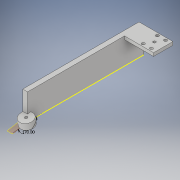
# Autodesk Inventor part: WheelIntakeMotorMount
Saved by Autodesk Inventor 2017 (Build 210142000, 142)
## iProperties
Created: 2017-11-15
Part Number: WheelIntakeMotorMount
Material: Generic
Document SubType Name: Modeling
Designer: User
Density: 1 g/cm^3
Appearance: Default
Author: User
Autodesk Inventor part; units mm, degrees
ref_plane "YZ Plane" through (0, 0, 0) normal (1, 0, 0) x (0, 1, 0)
ref_plane "XZ Plane" through (0, 0, 0) normal (0, 1, 0) x (-1, 0, 0)
ref_plane "XY Plane" through (0, 0, 0) normal (0, 0, 1) x (1, 0, 0)
sketch "Sketch2" plane through (0, 0, 0) normal (1, 0, 0) x (0, 1, 0)
  line L0 (0, 0) -> (25.4, 0)
  line L1 (25.4, 0) -> (25.4, -114.3)
  line L2 (25.4, -114.3) -> (0, -114.3)
  line L3 (0, -114.3) -> (0, 0)
  dimension "d6" = 25.4
  dimension "d7" = 114.3
  constraints: 8 end point, 2 parallel, 1 horizontal, 1 perpendicular
  measures "d6" distance of L1.end L2.end
  measures "d7" distance of L0.end L1.end
extrude "Extrusion2" add sketch "Sketch2" along normal blind 4.7625
sketch "Sketch3" plane through (4.7625, 0, 0) normal (1, 0, 0) x (0, 0, -1)
  line L0 (0, 0) -> (114.3, 0) projected
  line L1 (0, 0) -> (-14.429, -2.5442)
  line L2 (0, 0) -> (14.6516, 0) construction
  dimension "d10" = 170
  constraints: 4 end point, 1 equal length, 1 horizontal
  measures "d10" angle of L1 L2
ref_plane "Work Plane1" through (4.7625, -2.5442, 14.429) normal (0, 0.9848078, 0.1736482) x (0, 0.1736482, -0.9848078)
sketch "Sketch4" plane through (4.7625, -2.5442, 14.429) normal (0, 0.9848078, 0.1736482) x (0, 0.1736482, -0.9848078)
  line L0 (127.2151, 4.7625) -> (14.6516, 4.7625) projected
  line L1 (127.2151, 4.7625) -> (127.2151, 0) projected
  line L2 (14.6516, 0) -> (127.2151, 0) projected
  line L3 (14.6516, 4.7625) -> (14.6516, 0) projected
  line L4 (14.6516, 4.7625) -> (14.6516, 0)
  circle A0 centre (12.7466, -1.5875) radius 6.35
  dimension "d28" = 12.7
  dimension "d29" = 4.7625
  dimension "d30" = 1.5875
  dimension "d40" = 1.905
  constraints: 2 end point, 1 centre point, 1 collinear
  measures "d28" diameter of A0
  measures "d29" distance of L0.end L2.start
  measures "d30" distance from line of L2 A0.centre
  measures "d40" distance from line of A0.centre L3
sketch "Sketch5" plane through (0, 25.4, 0) normal (0, 1, 0) x (1, 0, 0)
  line L0 (0, 0) -> (0, 114.3) projected
  line L1 (0, 0) -> (4.7625, 0) projected
  line L2 (4.7625, 114.3) -> (4.7625, 0) projected
  line L3 (0, 114.3) -> (4.7625, 114.3) projected
  line L4 (0, 114.3) -> (0, 0) projected
  line L5 (0, 114.3) -> (33.3375, 114.3)
  line L6 (33.3375, 114.3) -> (33.3375, 95.25)
  line L7 (33.3375, 95.25) -> (0, 95.25)
  line L8 (0, 95.25) -> (0, 114.3)
  dimension "d47" = 33.3375
  dimension "d48" = 4.7625
  dimension "d49" = 19.05
  constraints: 8 end point, 2 parallel, 1 horizontal, 1 perpendicular
  measures "d47" distance of L6.end L7.end
  measures "d48" distance of L0.end L2.start
  measures "d49" distance of L5.end L6.end
extrude "Extrusion4" add sketch "Sketch5" against normal blind 3.175 contours L0 L3 L2 L7 | L2 L5 L6 L7
extrude "Extrusion6" add sketch "Sketch4" along normal blind 6.35 contours A0 L2 L3 | L3 L2 A0
sketch "Sketch10" plane through (0, 0, 0) normal (-1, 0, 0) x (0, 0, 1)
  line L0 (0, 25.4) -> (-114.3, 25.4) projected
  line L1 (-114.3, 25.4) -> (-114.3, 0) projected
  line L2 (-114.3, 0) -> (0, 0) projected
  line L3 (0, 0) -> (0, 25.4) projected
  line L4 (-3.0762, 6.9904) -> (-4.1789, 0.7369) projected
  line L5 (0, 6.448) -> (-3.0762, 6.9904) projected
  line L6 (0, 0) -> (0, 6.448) projected
  line L7 (-4.1789, 0.7369) -> (0, 0) projected
  line L8 (9.2323, 4.8201) -> (-3.2748, 7.0254) projected
  line L9 (8.1296, -1.4335) -> (9.2323, 4.8201) projected
  line L10 (3.078, 5.9052) -> (1.5105, -2.9848)
  line L11 (3.078, 5.9052) -> (12.1052, 5.9052) construction
  line L12 (-114.3, 0) -> (0, 0) projected
  line L13 (3.078, 5.9052) -> (0, 6.448)
  line L14 (0, 0) -> (0, 25.4) projected
  line L15 (0, 0) -> (0, 6.448)
  line L16 (0, 0) -> (1.9753, -0.3483)
  line L17 (5.253, -0.9262) -> (-1.5008, 0.2646) projected
  line L18 (0, 0) -> (4.9253, -0.8685)
  point P0 (-1.1172, 0.197)
  dimension "d41" = 12.3085
  dimension "d42" = 6.1542
  dimension "d43" = 100
  dimension "d44" = 8.89
  constraints: 12 end point, 4 point on line, 2 collinear, 1 equal length, 1 horizontal
  measures "d41" horizontal distance of L8.start L4.start
  measures "d42" horizontal distance of L8.start L10.start
  measures "d43" angle of L10 L11
  measures "d44" vertical distance of L10.start L10.end
extrude "Extrusion9" add sketch "Sketch10" against normal blind 2.54
sketch "Sketch11" plane through (0, 25.4, 0) normal (0, 1, 0) x (1, 0, 0)
  line L0 (0, 0) -> (4.7625, 0) projected
  line L1 (4.7625, 95.25) -> (4.7625, 0) projected
  line L2 (4.7625, 95.25) -> (33.3375, 95.25) projected
  line L3 (33.3375, 95.25) -> (33.3375, 114.3) projected
  line L4 (0, 114.3) -> (33.3375, 114.3) projected
  line L5 (0, 0) -> (0, 114.3) projected
  circle A0 centre (24.6375, 104.775) radius 8
  line L6 (20.6375, 111.7032) -> (28.6375, 111.7032)
  line L7 (28.6375, 111.7032) -> (28.6375, 97.8468)
  line L8 (28.6375, 97.8468) -> (20.6375, 97.8468)
  line L9 (20.6375, 97.8468) -> (20.6375, 111.7032)
  point P0 (0, 0)
  dimension "d50" = 16
  dimension "d53" = 19.05
  dimension "d54" = 28.575
  dimension "d55" = 9.525
  dimension "d56" = 8
  dimension "d57" = 4
  dimension "d58" = 15.875
  constraints: 8 end point, 4 coincident, 2 parallel, 2 point on circle, 1 centre point, 1 horizontal, 1 perpendicular
  measures "d50" diameter of A0
  measures "d53" distance of L2.end L3.end
  measures "d54" distance of L1.start L2.end
  measures "d55" distance from line of L4 A0.centre
  measures "d56" distance of L6.start L6.end
  measures "d57" distance from line of A0.centre L9
  measures "d58" distance from line of L1 point (20.637, 97.847)
hole "Hole1" at (20.6375, 25.4, -111.7032) at (28.6375, 25.4, -111.7032) at (28.6375, 25.4, -97.8468) at (20.6375, 25.4, -97.8468) direction (0, -1, 0) diameter 2.921 end through all
sketch "Sketch12" plane through (0, 25.4, 0) normal (0, 1, 0) x (1, 0, 0)
  circle A0 centre (28.6375, 97.8468) radius 1.4605 projected
  circle A1 centre (20.6375, 111.7032) radius 1.4605 projected
  circle A2 centre (28.6375, 111.7032) radius 1.4605 projected
  circle A3 centre (20.6375, 97.8468) radius 1.4605 projected
  line L0 (0, 0) -> (4.7625, 0) projected
  line L1 (4.7625, 95.25) -> (4.7625, 0) projected
  line L2 (4.7625, 95.25) -> (33.3375, 95.25) projected
  line L3 (33.3375, 95.25) -> (33.3375, 114.3) projected
  line L4 (0, 114.3) -> (33.3375, 114.3) projected
  line L5 (0, 0) -> (0, 114.3) projected
  circle A4 centre (28.6375, 97.8468) radius 1.4605 projected
  arc A5 (20.6375, 111.7032) -> (28.6375, 111.7032) centre (24.6375, 104.775) ccw
  point P0 (0, 0)
  constraints: 3 point on circle, 1 centre point
hole "Hole2" at (24.6375, 25.4, -104.775) direction (0, -1, 0) diameter 2.54 end through all
sketch "Sketch13" plane through (4.7625, 3.7093, 15.5317) normal (0, 0.9848078, 0.1736482) x (1, 0, 0)
  line L0 (-4.7625, 15.7713) -> (0, 15.7713) projected
  line L1 (-4.7625, 12.6458) -> (-4.7625, 15.7713) projected
  line L2 (-4.7625, 12.6458) -> (-4.7617, 12.6458) projected
  arc A0 (-4.7617, 12.6458) -> (0, 18.8949) centre (1.5875, 12.7466) ccw projected
  line L3 (0, 15.7713) -> (0, 18.8949) projected
  point P0 (-4.7625, 14.6516)
hole "Hole3" at (6.35, 5.9227, 2.9787) direction (0, -0.9848078, -0.1736482) diameter 2.54 end through all
equation "\"d30\" = 0.5 * d28 - d29"
equation "\"d42\" = 0.5 * d41"
equation "\"d55\" = 0.5 * d53"
equation "\"d57\" = 0.5 * d56"
body "Solid2"
